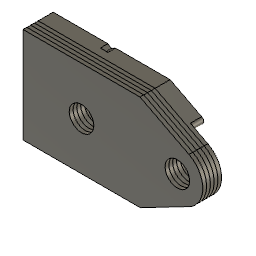
3-015 Reed Switch Mount (Autodesk Fusion 360 design; units mm, degrees)
Autodesk Fusion 360 part; units mm, degrees
sketch "Sketch1" plane through (0, 0, 0) normal (0, 1, 0) x (1, 0, 0)
  line L0 (0, 0) -> (0, -25.4)
  line L1 (0, 0) -> (27, 0)
  line L2 (-8, -24.4) -> (8, -24.4)
  line L3 (8, -24.4) -> (8, -21.9)
  line L4 (8, -21.9) -> (-8, -21.9)
  line L5 (-8, -21.9) -> (-8, -24.4) construction
  line L6 (-8, -23.15) -> (25.612717, -23.15) construction
  line L7 (8, -24.15) -> (14.5, -24.15)
  line L8 (14.5, -24.15) -> (14.5, -22.15)
  line L9 (14.5, -22.15) -> (8, -22.15)
  line L10 (14.5, -22.15) -> (14.5, 0)
  line L11 (9.5, -22.15) -> (9.5, 0)
  arc A0 (8.5, -22.15) -> (9.5, -21.15) centre (8.5, -21.15) ccw
  line L12 (9.5, -13.212836) -> (14.5, -13.212836) construction
  line L13 (12, -13.212836) -> (12, -15.774063) construction
  line L14 (0, -25.4) -> (15.5, -25.4)
  line L15 (15.5, -25.4) -> (15.5, 0)
  circle A1 centre (0, -12.7) radius 3.25
  line L16 (0, 0) -> (-21, 0) construction
  line L17 (-21, 0) -> (-21, -25.4) construction
  line L18 (-21, -25.4) -> (20, -25.4) construction
  circle A2 centre (25.4, -12.7) radius 3.25
  circle A3 centre (25.4, -12.7) radius 6.75
  line L19 (15.5, -25.4) -> (28.493754, -18.699265)
  line L20 (15.5, 0) -> (28.493754, -6.700735)
  circle A4 centre (0, -12.7) radius 6.75
  line L21 (0, -24.8) -> (1, -25.4)
  point P0 (0, -21.9)
  dimension "d1" = 16
  dimension "d2" = 2.5
  dimension "d3" = 2
  dimension "d4" = 5
  dimension "d5" = 12
  dimension "d6" = 1
  dimension "d7" = 1
  dimension "d8" = 1
  dimension "d9" = 6.5
  dimension "d10" = 25.4
  dimension "d11" = 3.5
  dimension "d34" = 25.4
  dimension "d35" = 1
  dimension "d36" = 0.4
  constraint coincident L0.start L1.start
  constraint vertical L0
  constraint perpendicular L0 L1
  constraint horizontal L2
  constraint vertical L3
  constraint horizontal L4
  constraint vertical L5
  constraint midpoint L4 P0
  constraint coincident L0 P0
  constraint midpoint L5 L6.start
  constraint perpendicular L5 L6
  constraint coincident L3 L7.start
  constraint perpendicular L3 L7
  constraint perpendicular L6 L8
  constraint coincident L3 L9.end
  constraint perpendicular L3 L9
  constraint symmetric L6 L7 L9
  constraint coincident L1 L10.end
  constraint perpendicular L1 L10
  constraint coincident L9 L11.start
  constraint coincident L1 L11.end
  constraint perpendicular L1 L11
  constraint tangent L11 A0
  constraint coincident L11 A0.end
  constraint coincident L9 A0.start
  constraint tangent L9 A0
  constraint perpendicular L10 L12
  constraint perpendicular L12 L13
  constraint coincident L0 L14.start
  constraint perpendicular L0 L14
  constraint coincident L1 L15.end
  constraint perpendicular L1 L15
  constraint coincident L0 A1.centre
  constraint perpendicular L0 L16
  constraint perpendicular L16 L17
  constraint perpendicular L0 L18
  constraint coincident L0.end L18
  constraint equal A1 A2
  constraint horizontal A1.centre A2.centre
  constraint concentric A2 A3
  constraint tangent A3 L19
  constraint midpoint L0 A1.centre
  constraint tangent A3 L20
  constraint concentric A1 A4
  constraint equal A3 A4
  constraint coincident L0 L21.start
  constraint coincident L18 L21.end
  measures "d1" distance of L2.start L2.end
  measures "d2" distance of L2.end L3.end
  measures "d3" distance of L7.end L8.end
  measures "d4" distance of L10 L11
  measures "d5" distance of L0 L13
  measures "d6" radius of A0
  measures "d7" distance of L10 L15
  measures "d8" distance of L2 L14
  measures "d9" diameter of A1
  measures "d10" distance of L16.end L17.end
  measures "d11" distance of A2 A3
  measures "d34" distance of A2.centre A1.centre
  measures "d35" distance of L0 L21.end
  measures "d36" distance of L2 L21.start
extrude "Extrude1" add sketch "Sketch1" along normal blind 4 contours L0 L14 L21 | L0 L1 L2 L3 L7 L8 L10 L14 L15 L21 | L0 L2 L3 L4 | L0 L1 L3 L4 L9 L11 A0 A4 | L0 A1 A4 | L3 L7 L8 L9 | L1 L9 L10 L11 | L9 L11 A0 picked at (0.333333, -25.2) picked at (12.666667, -24.65) picked at (2.666667, -22.816667) picked at (4.10135, -2.186661) picked at (5.549405, -13.174383) picked at (10.666667, -23.483333) picked at (12.833333, -14.433333) picked at (9.303537, -21.953537) makes body 1
extrude "Extrude2" cut sketch "Sketch1" along normal blind 3 contours L0 L2 L3 L4 | L3 L7 L8 L9 | L1 L9 L10 L11 | L9 L11 A0 picked at (2.666667, -22.816667) picked at (10.666667, -23.483333) picked at (12.833333, -14.433333) picked at (9.303537, -21.953537) bodies 1
extrude "Extrude3" add sketch "Sketch1" against normal blind 1 separate body contours L0 L14 L21 | L0 L1 L2 L3 L7 L8 L10 L14 L15 L21 | L0 L2 L3 L4 | L0 L1 L3 L4 L9 L11 A0 A4 | L0 A1 A4 | L3 L7 L8 L9 | L1 L9 L10 L11 | L9 L11 A0 picked at (0.333333, -25.2) picked at (12.666667, -24.65) picked at (2.666667, -22.816667) picked at (4.10135, -2.186661) picked at (5.549405, -13.174383) picked at (10.666667, -23.483333) picked at (12.833333, -14.433333) picked at (9.303537, -21.953537) makes body 2
extrude "Extrude4" cut sketch "Sketch1" against normal up to surface (3 mm away) from surface at 4 contours L0 A1 A4 picked at (5.549405, -13.174383) bodies 1
extrude "Extrude8" cut sketch "Sketch1" against normal blind 2 from surface at 4 contours L0 L14 L21 picked at (0.333333, -25.2) bodies 1
mirror "Mirror1" about plane through (0, 0, 0) normal (1, 0, 0) of bodies 1 merged
mirror "Mirror2" about plane through (0, 0, 0) normal (1, 0, 0) of bodies 2 merged
extrude "Extrude5" add sketch "Sketch1" along normal up to surface (4 mm away) separate body contours L15 A3 L19 L20 picked at (16.55, -12.7) makes body 3
extrude "Extrude6" add sketch "Sketch1" along normal up to surface (1 mm away) contours A3 picked at (27.555946, -17.836861) bodies 3
fillet "Fillet1" radius 1 2 edges at (28.493754, 2.5, 18.699265) (28.493754, 2.5, 6.700735) on bodies 3
extrude "Extrude7" add sketch "Sketch1" against normal up to surface (0.9998 mm away) contours L15 A3 L19 L20 | A3 picked at (16.55, -12.7) picked at (27.555946, -17.836861) bodies 2
combine "Combine1" operation add target body 1 tool bodies 3
copy_body "Body->Comp1" bodies 1 removing the originals makes body 4 in component "Top Housing"
copy_body "Body->Comp2" bodies 2 removing the originals makes body 5 in component "Back Plate"
component "Top Housing" placed x (1, 0, 0) y (0, 1, 0) z (0, 0, 1) at (0, 0, 0)
component "Back Plate" placed x (1, 0, 0) y (0, 1, 0) z (0, 0, 1) at (0, 0, 0)
component "Back Plate" placed x (1, 0, 0) y (0, 1, 0) z (0, 0, 1) at (0, -1, 0)
component "Back Plate" placed x (1, 0, 0) y (0, 1, 0) z (0, 0, 1) at (0, -2, 0)
component "Back Plate" placed x (1, 0, 0) y (0, 1, 0) z (0, 0, 1) at (0, -3, 0)
equation "d5 = ( 24 / 2 ) * 1 mm"
equation "d7 = d8"
named bodies: "Top Housing", "Back Plate"
